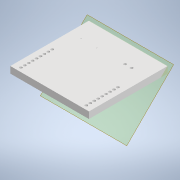
# Autodesk Inventor part: Деталь7
Saved by Autodesk Inventor 2021.2 (Build 252289000, 289)
## iProperties
Created: 2022-10-18
Part Number: Деталь7
Material: Типовые
Document SubType Name: Modeling
Designer: 22-91-12
Density: 1 g/cm^3
Appearance: По умолчанию
Author: 22-91-12
Autodesk Inventor part; units mm, degrees
ref_plane "YZ Plane" through (0, 0, 0) normal (1, 0, 0) x (0, 1, 0)
ref_plane "XZ Plane" through (0, 0, 0) normal (0, 1, 0) x (-1, 0, 0)
ref_plane "XY Plane" through (0, 0, 0) normal (0, 0, 1) x (1, 0, 0)
sketch "Эскиз1" plane through (0, 0, 0) normal (0, 1, 0) x (-1, 0, 0)
  line L0 (0, 30) -> (30, 30)
  line L1 (30, 30) -> (30, -30)
  line L2 (30, -30) -> (-20, -30)
  line L3 (-20, 30) -> (0, 30)
  line L4 (-30, 0) -> (-30, -30)
  line L5 (-30, -30) -> (-30, 30)
  line L6 (-20, 30) -> (-30, 30)
  line L7 (-30, -30) -> (-20, -30)
  point P0 (0, 0)
  constraints: 16 end point, 4 point on line, 2 perpendicular
extrude "Выдавливание1" add sketch "Эскиз1" along normal blind 5
sketch "Эскиз2" plane through (0, 5, 0) normal (0, 1, 0) x (1, 0, 0)
  line L0 (-30, 30) -> (-30, -30) projected
  line L1 (-30, 0) -> (30, 0)
  line L2 (30, -30) -> (30, 30) projected
  line L3 (0, 0) -> (0, 30)
  line L4 (30, 30) -> (-30, 30) projected
  line L5 (0, 15) -> (30, 15)
  line L6 (15, 0) -> (15, 30)
  line L7 (15, 15) -> (12.5, 15)
  line L8 (12.5, 15) -> (17.5, 15)
  dimension "d46" = 2.5
  dimension "d47" = 5
  constraints: 12 end point, 5 midpoint, 5 point on line, 2 perpendicular
  measures "d46" distance of L7.start L7.end
  measures "d47" distance of L7.end L8.end
sketch "Эскиз3" plane through (0, 5, 0) normal (0, 1, 0) x (1, 0, 0)
  line L0 (30, -30) -> (30, 30) projected
  line L1 (-30, -30) -> (30, -30) projected
  line L2 (25, 0) -> (25, -3)
  line L3 (25, -30) -> (25, -27)
  line L4 (-25, -27) -> (-25, -3)
  line L5 (-25, -27) -> (-25, -24)
  line L6 (-25, -24) -> (-25, -21)
  line L7 (-25, -21) -> (-25, -18)
  line L8 (-25, -18) -> (-25, -15)
  line L9 (-25, -15) -> (-25, -12)
  line L10 (-25, -12) -> (-25, -9)
  line L11 (-25, -9) -> (-25, -6)
  line L12 (25, -27) -> (25, -3)
  line L13 (25, -27) -> (25, -24)
  line L14 (25, -24) -> (25, -21)
  line L15 (25, -21) -> (25, -18)
  line L16 (25, -18) -> (25, -15)
  line L17 (25, -15) -> (25, -12)
  line L18 (25, -12) -> (25, -9)
  line L19 (25, -9) -> (25, -6)
  point P0 (0, 0)
  dimension "d19" = 3
  dimension "d20" = 3
  dimension "d21" = 3
  dimension "d22" = 3
  dimension "d23" = 3
  dimension "d24" = 3
  dimension "d25" = 3
  dimension "d26" = 3
  dimension "d27" = 3
  dimension "d28" = 3
  constraints: 32 end point, 1 point on line, 20 other
  measures "d19" distance of L5.start L5.end
  measures "d20" distance of L5.end L6.end
  measures "d21" distance of L6.end L7.end
  measures "d22" distance of L7.end L8.end
  measures "d23" distance of L8.end L9.end
  measures "d24" distance of L9.end L10.end
  measures "d25" distance of L10.end L11.end
  measures "d26" distance of L3.end L13.end
  measures "d27" distance of L13.end L14.end
  measures "d28" distance of L14.end L15.end
hole "Отверстие1" at (-25, 5, 27) at (-25, 5, 24) at (-25, 5, 21) at (-25, 5, 18) at (-25, 5, 15) at (-25, 5, 12) at (-25, 5, 9) at (-25, 5, 6) at (-25, 5, 3) at (25, 5, 27) at (25, 5, 24) at (25, 5, 21) at (25, 5, 18) at (25, 5, 15) at (25, 5, 12) at (25, 5, 9) at (25, 5, 6) at (25, 5, 3) direction (0, -1, 0) diameter 2 end through all
sketch "Эскиз4" plane through (0, 5, 0) normal (0, 1, 0) x (1, 0, 0)
  line L0 (-30, 30) -> (-30, -30) projected
  line L1 (-30, 0) -> (-30, 15)
  line L2 (-30, 15) -> (0, 15)
  line L3 (-30, 15) -> (-21, 15)
  line L4 (0, 15) -> (-9, 15)
  point P0 (0, 0)
  dimension "d36" = 15
  dimension "d37" = 9
  dimension "d38" = 9
  constraints: 8 end point, 3 point on line, 1 midpoint, 1 perpendicular
  measures "d36" distance of L1.start L1.end
  measures "d37" distance of L1.end L3.end
  measures "d38" distance of L2.end L4.end
hole "Отверстие2" at (-21, 5, -15) at (-9, 5, -15) direction (0, -1, 0) diameter 0.7 end through all
hole "Отверстие3" at (12.5, 5, -15) at (17.5, 5, -15) direction (0, -1, 0) diameter 2 end through all
ref_plane "РабПлоскость1" through (30, 5, -30) normal (0, -0.7071, -0.7071) x (-1, 0, 0)
